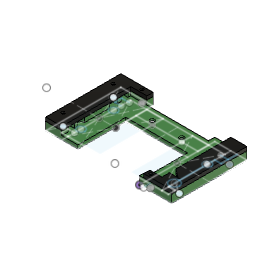
Mounting Brackets v7 (Autodesk Fusion 360 design; units mm, degrees)
Autodesk Fusion 360 part; units mm, degrees
sketch "Sketch1" plane through (0, 0, 0) normal (0, 0, 1) x (1, 0, 0)
  line L0 (0, 0) -> (60, 0)
  line L1 (60, 0) -> (60, 140)
  line L2 (60, 140) -> (0, 140)
  line L3 (0, 140) -> (0, 0)
  line L4 (0, 70) -> (60, 70) construction
  line L5 (-30, 11.5) -> (30, 11.5)
  line L6 (30, 11.5) -> (30, 128.5)
  line L7 (30, 128.5) -> (-30, 128.5)
  line L8 (-30, 128.5) -> (-30, 11.5)
  line L9 (-30, 11.5) -> (30, 128.5) construction
  line L10 (30, 11.5) -> (-30, 128.5) construction
  line L11 (30, 11.5) -> (42, 11.5)
  line L12 (42, 11.5) -> (42, 23.5)
  line L13 (42, 23.5) -> (30, 23.5)
  line L14 (30, 23.5) -> (30, 25.5)
  line L15 (30, 25.5) -> (46, 25.5)
  line L16 (30, 25.5) -> (30, 37.5)
  line L17 (30, 37.5) -> (46, 25.5)
  circle A0 centre (29.5925, 35.2951) radius 9
  line L18 (29.5925, 35.2951) -> (29.5925, 110.2951)
  line L19 (29.5925, 110.2951) -> (41.5925, 110.2951)
  line L20 (41.5925, 110.2951) -> (41.5925, 123.2951)
  line L21 (41.5925, 123.2951) -> (27.5925, 123.2951)
  line L22 (29.5925, 110.2951) -> (29.5925, 95.8151) construction
  line L23 (29.5925, 96.5614) -> (27.6225, 96.5614)
  circle A1 centre (29.8335, 96.4112) radius 7
  line L24 (41.5925, 116.7951) -> (60, 116.7951) construction
  line L25 (41.5925, 123.2951) -> (41.5925, 140)
  circle A2 centre (50.7963, 116.7951) radius 1.75
  circle A3 centre (50.7963, 23.2049) radius 1.75
  line L26 (0, 128.5) -> (-115, 128.5)
  line L27 (-115, 128.5) -> (-115, 108.5)
  line L28 (-115, 108.5) -> (0, 108.5)
  line L29 (0, 108.5) -> (0, 128.5)
  line L30 (0, 70) -> (-243.4546, 70) construction
  line L31 (-115, 108.5) -> (-115, 70)
  line L32 (-85, 11.5) -> (-145, 11.5)
  line L33 (-145, 11.5) -> (-145, 128.5)
  line L34 (-145, 128.5) -> (-85, 128.5)
  line L35 (-85, 128.5) -> (-85, 11.5)
  line L36 (-85, 11.5) -> (-145, 128.5) construction
  line L37 (-145, 11.5) -> (-85, 128.5) construction
  line L38 (-57.5, 128.5) -> (-57.5, 11.4304) construction
  circle A4 centre (-144.8335, 96.4112) radius 7
  line L39 (-115, 0) -> (-175, 0)
  line L40 (-175, 0) -> (-175, 140)
  line L41 (-175, 140) -> (-115, 140)
  line L42 (-115, 140) -> (-115, 0)
  line L43 (-115, 0) -> (-175, 140) construction
  line L44 (-175, 0) -> (-115, 140) construction
  circle A5 centre (-165.7963, 23.2049) radius 1.75
  line L45 (-157, 11.5) -> (-157, 23.5)
  line L46 (-157, 23.5) -> (-145, 23.5)
  line L47 (-145, 11.5) -> (-157, 11.5)
  line L48 (-156.5925, 123.2951) -> (-142.5925, 123.2951)
  line L49 (-144.5925, 110.2951) -> (-156.5925, 110.2951)
  line L50 (-156.5925, 110.2951) -> (-156.5925, 123.2951)
  line L51 (-115, 89.25) -> (0, 89.25)
  circle A6 centre (-165.7963, 116.7951) radius 1.75
  circle A7 centre (-85, 108.5) radius 2.75
  circle A8 centre (-30, 108.5) radius 2.75
  line L52 (-145, 11.5) -> (-145, 0)
  line L53 (-115, 140) -> (-130, 140) construction
  line L54 (-130, 140) -> (-130, 128.5) construction
  circle A9 centre (-130, 134.25) radius 1.75
  line L55 (0, 0) -> (15, 0) construction
  line L56 (15, 0) -> (15, 11.5) construction
  circle A10 centre (15, 5.75) radius 1.75
  line L57 (30, 128.5) -> (30, 140)
  circle A11 centre (-130, 134.25) radius 3
  circle A12 centre (15, 5.75) radius 3.25
  circle A13 centre (50.7963, 116.7951) radius 3.25
  circle A14 centre (50.7963, 23.2049) radius 3.25
  circle A15 centre (-165.7963, 116.7951) radius 3.25
  circle A16 centre (-165.7963, 23.2049) radius 3.25
  line L58 (7.576, 11.5) -> (7.576, 0)
  circle A17 centre (-144.5925, 35.2951) radius 7
  circle A18 centre (50.7963, 116.7951) radius 2.5
  circle A19 centre (50.7963, 23.2049) radius 2.5
  circle A20 centre (15, 5.75) radius 2.5
  circle A21 centre (-130, 134.25) radius 2.5
  circle A22 centre (-165.7963, 116.7951) radius 2.5
  circle A23 centre (-165.7963, 23.2049) radius 2.5
  point P0 (0, 70)
  point P1 (-115, 70)
  point P2 (-145, 70)
  point P3 (-165.7963, 116.7951)
  dimension "d1" = 60
  dimension "d2" = 140
  dimension "d3" = 60
  dimension "d4" = 117
  dimension "d5" = 12
  dimension "d6" = 12
  dimension "d7" = 2
  dimension "d8" = 16
  dimension "d9" = 12
  dimension "d11" = 18
  dimension "d12" = 75
  dimension "d13" = 12
  dimension "d14" = 13
  dimension "d15" = 14
  dimension "d17" = 14.48
  dimension "d18" = 1.97
  dimension "d20" = 14
  dimension "d27" = 3.5
  dimension "d31" = 115
  dimension "d32" = 20
  dimension "d33" = 60
  dimension "d34" = 117
  dimension "d35" = 60
  dimension "d36" = 140
  dimension "d44" = 5.5
  dimension "d53" = 15
  dimension "d54" = 3.5
  dimension "d55" = 15
  dimension "d56" = 3.5
  dimension "d64" = 12
  dimension "d65" = 6
  dimension "d66" = 6.5
  dimension "d67" = 6.5
  dimension "d68" = 6.5
  dimension "d72" = 6.5
  dimension "d73" = 6.5
  dimension "d80" = 14
  dimension "d81" = 5
  dimension "d82" = 5
  dimension "d83" = 5
  dimension "d84" = 5
  dimension "d85" = 5
  dimension "d86" = 5
  constraint horizontal L0
  constraint vertical L1
  constraint horizontal L2
  constraint vertical L3
  constraint coincident L0.start L3.end
  constraint midpoint L3 P0
  constraint midpoint L1 L4.end
  constraint horizontal L5
  constraint perpendicular L5 L6
  constraint parallel L5 L7
  constraint parallel L6 L8
  constraint coincident L9 P0
  constraint coincident L10 P0
  constraint coincident P0 L4.start
  constraint perpendicular L6 L11
  constraint perpendicular L11 L12
  constraint coincident L6 L13.end
  constraint perpendicular L6 L13
  constraint coincident L6 L14.end
  constraint perpendicular L6 L15
  constraint perpendicular L15 L16
  constraint coincident A0.centre L18.start
  constraint parallel L6 L18
  constraint perpendicular L18 L19
  constraint perpendicular L19 L20
  constraint perpendicular L6 L21
  constraint perpendicular L19 L22
  constraint coincident L22 L23.start
  constraint perpendicular L22 L23
  constraint midpoint L20 L24.start
  constraint coincident L1 L24.end
  constraint perpendicular L1 L24
  constraint coincident L2 L25.end
  constraint perpendicular L2 L25
  constraint midpoint L24 A2.centre
  constraint symmetric L4 A2 A3
  constraint horizontal L26
  constraint vertical L27
  constraint horizontal L28
  constraint vertical L29
  constraint midpoint L7 L26.start
  constraint parallel L4 L30
  constraint coincident L30 P1
  constraint perpendicular L30 L31
  constraint horizontal L32
  constraint perpendicular L32 L33
  constraint parallel L32 L34
  constraint parallel L33 L35
  constraint coincident L36 P1
  constraint coincident L37 P1
  constraint coincident P1 L31.end
  constraint midpoint L26 L38.start
  constraint perpendicular L26 L38
  constraint symmetric A1 L38 A4
  constraint horizontal L39
  constraint perpendicular L39 L40
  constraint parallel L39 L41
  constraint parallel L40 L42
  constraint coincident L43 P2
  constraint coincident L44 P2
  constraint midpoint L33 P2
  constraint symmetric L5.end L38 L32.end
  constraint symmetric L11.end L38 L45.start
  constraint symmetric L12.end L38 L45.end
  constraint symmetric L13.end L38 L46.end
  constraint symmetric A2.centre L38 P3
  constraint symmetric A3 L38 A5
  constraint symmetric L18.end L38 L49.start
  constraint symmetric L19.end L38 L49.end
  constraint symmetric L20.end L38 L48.start
  constraint symmetric L21.end L38 L48.end
  constraint midpoint L31 L51.start
  constraint coincident L3 L51.end
  constraint perpendicular L3 L51
  constraint symmetric A2 L38 A6
  constraint coincident L35 A7.centre
  constraint coincident L28 A7.centre
  constraint symmetric L38 A7 A8
  constraint midpoint L39 L52.end
  constraint perpendicular L42 L53
  constraint coincident L34 L54.end
  constraint perpendicular L34 L54
  constraint midpoint L54 A9.centre
  constraint perpendicular L3 L55
  constraint coincident L5 L56.end
  constraint perpendicular L5 L56
  constraint midpoint L56 A10.centre
  constraint midpoint L2 L57.end
  constraint concentric A9 A11
  constraint concentric A10 A12
  constraint concentric A2 A13
  constraint concentric A3 A14
  constraint concentric A6 A15
  constraint concentric A5 A16
  constraint coincident L5 L58.start
  constraint perpendicular L5 L58
  constraint concentric A13 A18
  constraint concentric A14 A19
  constraint concentric A10 A20
  constraint concentric A11 A21
  constraint concentric A6 A22
  constraint concentric A16 A23
  measures "d1" distance of L0.start L0.end
  measures "d2" distance of L0.start L2.end
  measures "d3" distance of L6.end L7.end
  measures "d4" distance of L5.end L6.end
  measures "d5" distance of L5.end L11.end
  measures "d6" distance of L11.end L12.end
  measures "d7" distance of L13.end L14.end
  measures "d8" distance of L14.end L15.end
  measures "d9" distance of L14.end L16.end
  measures "d11" diameter of A0
  measures "d12" distance of A0.centre L18.end
  measures "d13" distance of L18.end L19.end
  measures "d14" distance of L19.end L20.end
  measures "d15" distance of L20.end L21.end
  measures "d17" distance of L18.end L22.end
  measures "d18" distance of L23.start L23.end
  measures "d20" diameter of A1
  measures "d27" diameter of A2
  measures "d31" distance of L26.start L26.end
  measures "d32" distance of L26.start L28.end
  measures "d33" distance of L33.end L34.end
  measures "d34" distance of L32.end L33.end
  measures "d35" distance of L40.end L41.end
  measures "d36" distance of L39.end L40.end
  measures "d44" diameter of A7
  measures "d53" distance of L41.end L53.end
  measures "d54" diameter of A9
  measures "d55" distance of L0.start L55.end
  measures "d56" diameter of A10
  measures "d64" distance of L45.start L32.end
  measures "d65" diameter of A11
  measures "d66" diameter of A12
  measures "d67" diameter of A13
  measures "d68" diameter of A14
  measures "d72" diameter of A15
  measures "d73" diameter of A16
  measures "d80" diameter of A17
  measures "d81" diameter of A18
  measures "d82" diameter of A19
  measures "d83" diameter of A20
  measures "d84" diameter of A21
  measures "d85" diameter of A22
  measures "d86" diameter of A23
extrude "Extrude1" add sketch "Sketch1" along normal blind 7 contours L0 L3 L5 L58 | L0 L1 L2 L5 L6 L11 L12 L13 L14 L15 L17 A0 L19 L20 A1 L25 L58 | L3 L5 L6 L7 L14 L16 A0 L18 L19 A1 L29 | L6 L11 L12 L13 | L2 L6 L21 L25 L57 | L2 L3 L7 L57 | L6 L19 L20 L21 | L6 L15 L16 L17 A0 | L6 L16 A0 | L6 L16 L17 A0 | L6 L18 L19 A1 | L6 L17 A0 | L6 A0 L18 A1 | L6 A1 | L6 L18 A1 | L18 A1 | A2 | A3 | A10 | A12 | A13 | A14 | A18 | A19 | A20 makes body 1
extrude "Extrude2" add sketch "Sketch1" along normal blind 8 from surface at 7 contours L0 L3 L5 L58 | L0 L1 L2 L5 L6 L11 L12 L13 L14 L15 L17 A0 L19 L20 A1 L25 L58 | L2 L6 L21 L25 L57 | A2 | A3 | A10 | A12 | A13 | A14 | A18 | A19 | A20 bodies 1
extrude "Extrude3" cut sketch "Sketch1" against normal blind 6 from surface at 15 contours A2 | A3 | A10 | A18 | A19 | A20 bodies 1
extrude "Extrude4" add sketch "Sketch1" along normal blind 7 separate body contours L27 L31 L32 L33 L34 A4 L42 A17 | L32 L39 L42 L52 | L33 L34 A4 L39 L40 L41 L42 L45 L46 L47 L48 L49 L50 L52 A17 | L33 L45 L46 L47 | L33 L48 L49 L50 | L33 A17 | L33 A17 | L33 A4 | L33 A4 | A5 | A6 | A9 | A11 | A15 | A16 | A21 | A22 | A23 makes body 2
extrude "Extrude5" add sketch "Sketch1" along normal blind 8 from surface at 7 contours L33 L34 A4 L39 L40 L41 L42 L45 L46 L47 L48 L49 L50 L52 A17 | A5 | A6 | A9 | A11 | A15 | A16 | A21 | A22 | A23 bodies 2
extrude "Extrude6" add sketch "Sketch1" along normal blind 7 contours L3 L8 L28 L51 A8 | L3 L7 L8 L26 L28 L29 A8 | L8 L28 L35 L51 A7 A8 | L8 L28 A8 | L8 L28 A8 | L8 L28 A8 | L28 L31 L35 L42 L51 A7 | L8 L26 L28 L35 A7 A8 | L8 L28 A8 | L28 L35 A7 | L28 L35 A7 | L26 L27 L28 L34 L35 L42 A7 | L28 L35 A7 | L28 L35 A7 bodies 1 2
extrude "Extrude7" cut sketch "Sketch1" along normal up to surface (7 mm away) contours L8 L28 A8 | L8 L28 A8 | L8 L28 A8 | L8 L28 A8 | L28 L35 A7 | L28 L35 A7 | L28 L35 A7 | L28 L35 A7 bodies 1
extrude "Extrude12" cut sketch "Sketch1" against normal blind 8 from surface at 15 contours A5 | A6 | A9 | A21 | A22 | A23 bodies 1
extrude "Extrude8" add sketch "Sketch1" along normal blind 7 from surface at 15 separate body contours L0 L1 L2 L5 L6 L11 L12 L13 L14 L15 L17 A0 L19 L20 A1 L25 L58 | L6 L11 L12 L13 | L2 L6 L21 L25 L57 | L6 L19 L20 L21 | L6 L17 A0 | L6 A1 | A12 | A13 | A14 | A18 | A19 | A20 makes body 3
chamfer "Chamfer2" distance 1.5 angle 45 2 edges at (-87.5639, 109.4944, 7) (-32.5639, 109.4944, 7) on bodies 1
extrude "Extrude9" add sketch "Sketch1" along normal blind 7 from surface at 15 separate body contours L33 L34 A4 L39 L40 L41 L42 L45 L46 L47 L48 L49 L50 L52 A17 | L33 L45 L46 L47 | L33 L48 L49 L50 | L33 A17 | L33 A4 | A11 | A15 | A16 | A21 | A22 | A23 picked at (-147.0478, 36.1173) picked at (-148.7889, 95.4398) makes body 4
extrude "Extrude10" cut sketch "Sketch1" against normal blind 3 from surface at 22 contours A12 | A13 | A14 | A18 | A19 | A20 bodies 3
extrude "Extrude11" cut sketch "Sketch1" against normal blind 3 from surface at 22 contours A11 | A15 | A16 | A21 | A22 | A23 bodies 4
named bodies: "Back", "Left Side", "Right Side"
